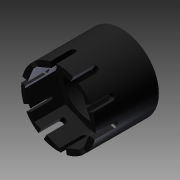
# Autodesk Inventor part: Spindle for Fisher Gearbox
Saved by Autodesk Inventor 2011 (Build 150239000, 239)
## iProperties
Shininess: 64.0
Angle Display Precision: 2
Document Length Units: 11272
Document Angle Units: 11279
Document Time Units: 11290
Document Mass Units: 11286
Document Length Units Precision: 3
Document Angle Units Precision: 2
Category: Motors
Created: 2001-12-28
Document SubType Name: Modeling
Density: 1 g/cm^3
Project: FIRST
Vendor: Fisher
Description: Spindle for Fisher Gearbox
Density: 0.0
Volumn: 0.0
Area: 0.0
PropertySet Name: Model Information
Control State: 0
Master: False
Checked Out: False
Title: Spindle for Fisher Gearbox
Author: Autodesk, Inc.
Autodesk Inventor part; units mm, degrees
ref_plane "YZ Plane" through (0, 0, 0) normal (1, 0, 0) x (0, 1, 0)
ref_plane "XZ Plane" through (0, 0, 0) normal (0, 1, 0) x (-1, 0, 0)
ref_plane "XY Plane" through (0, 0, 0) normal (0, 0, 1) x (1, 0, 0)
sketch "Sketch1" plane through (0, 0, 0) normal (0, 0, 1) x (1, 0, 0)
  circle A0 centre (57.9029, 21.7713) radius 22.606
  dimension "d0" = 45.212
  constraints: 1 centre point
  measures "d0" diameter of A0
extrude "Extrusion1" add sketch "Sketch1" along normal blind 38.1
sketch "Sketch2" plane through (57.9029, 21.7713, 38.1) normal (0, 0, 1) x (1, 0, 0)
  circle A0 centre (0, 0) radius 22.606 projected
  circle A1 centre (0, 0) radius 15.875
  dimension "d3" = 31.75
  constraints: 1 centre point, 1 coincident
  measures "d3" diameter of A1
extrude "Extrusion2" cut sketch "Sketch2" against normal blind 38.1 contours A1
sketch "Sketch3" plane through (57.9029, 21.7713, 38.1) normal (0, 0, 1) x (1, 0, 0)
  circle A0 centre (0, 0) radius 15.875 projected
  circle A1 centre (0, 0) radius 22.606 projected
  line L0 (-20.6196, 0) -> (-14.5802, 14.5802)
  line L1 (-14.5802, 14.5802) -> (0, 20.6196)
  line L2 (0, 20.6196) -> (14.5802, 14.5802)
  line L3 (14.5802, 14.5802) -> (20.6196, 0)
  line L4 (20.6196, 0) -> (14.5802, -14.5802)
  line L5 (14.5802, -14.5802) -> (0, -20.6196)
  line L6 (0, -20.6196) -> (-14.5802, -14.5802)
  line L7 (-14.5802, -14.5802) -> (-20.6196, 0)
  dimension "d6" = 38.1
  constraints: 16 end point, 1 coincident, 15 other
  measures "d6" distance between parallel lines of L0 L4
extrude "Extrusion3" cut sketch "Sketch3" against normal blind 18.796 contours L0 L1 L2 L3 L4 L5 L6 L7
sketch "Sketch4" plane through (57.9029, 21.7713, 38.1) normal (0, 0, 1) x (1, 0, 0)
  line L0 (0, 20.6196) -> (14.5802, 14.5802) projected
  circle A0 centre (0, 0) radius 22.606 projected
  line L1 (0, 0) -> (15.2644, 28.8495)
  line L2 (7.2987, 17.5963) -> (8.9679, 20.7511)
  line L3 (10.5986, 16.2295) -> (12.1111, 19.088)
  dimension "d9" = 3.556
  constraints: 6 end point, 2 point on circle, 2 point on line, 1 other
  measures "d9" diameter of L2 L1
extrude "Extrusion4" cut sketch "Sketch4" against normal blind 13.462 contours L2 A0 L1 L0 | L1 A0 L3 L0
fillet "Fillet1" radius 1.651 2 edges at (69.2577, 39.4301, 24.638) (66.0362, 40.945, 24.638)
pattern_circular "Circular Pattern1" count 10 over 360 about axis through (57.9029, 21.7713, 0) along (0, 0, 1) of "Extrusion4", "Fillet1"
body "Solid1"
